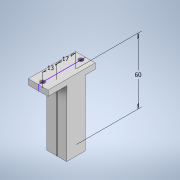
# Autodesk Inventor part: AdaptadorAnycubic
Saved by Autodesk Inventor 2020.3 (Build 243373000, 373)
## iProperties
Created: 2020-08-24
Part Number: AdaptadorAnycubic
Material: Generic
Document SubType Name: Modeling
Designer: mifer
Density: 1 g/cm^3
Appearance: Default
Author: mifer
Autodesk Inventor part; units mm, degrees
ref_plane "YZ Plane" through (0, 0, 0) normal (1, 0, 0) x (0, 1, 0)
ref_plane "XZ Plane" through (0, 0, 0) normal (0, 1, 0) x (-1, 0, 0)
ref_plane "XY Plane" through (0, 0, 0) normal (0, 0, 1) x (1, 0, 0)
sketch "Sketch1" plane through (0, 0, 0) normal (1, 0, 0) x (0, 1, 0)
  line L0 (0, 0) -> (-60, 0)
  line L1 (-60, 0) -> (-60, -17)
  line L2 (-60, -17) -> (0, -17)
  line L3 (0, -17) -> (0, 0)
  line L4 (0, -22) -> (5, -22)
  line L5 (5, -22) -> (5, 13)
  line L6 (5, 13) -> (0, 13)
  line L7 (0, 13) -> (0, -22)
  line L8 (5, 13) -> (0, 13)
  line L9 (0, 13) -> (0, 17)
  line L10 (0, 17) -> (5, 17)
  line L11 (5, 17) -> (5, 13)
  line L12 (5, -22) -> (0, -22)
  line L13 (0, -22) -> (0, -26)
  line L14 (0, -26) -> (5, -26)
  line L15 (5, -26) -> (5, -22)
  point P0 (0, 13)
  point P1 (0, -17)
  dimension "d0" = 17
  dimension "d1" = 60
  dimension "d2" = 13
  constraints: 32 end point, 8 parallel, 4 horizontal, 4 perpendicular, 1 point on line
  measures "d0" distance of L2.end L0.start
  measures "d1" distance of L1.end L2.end
  measures "d2" distance of L0.start L6.end
extrude "Extrusion1" add sketch "Sketch1" along normal mid plane 18
sketch "Sketch2" plane through (-9, 5, 17) normal (0, 1, 0) x (1, 0, 0)
  circle A0 centre (9, 39) radius 2
  circle A1 centre (9, 4) radius 2
  point P0 (9, 17)
  dimension "d5" = 4
  dimension "d6" = 4
  constraints: 2 centre point
  measures "d5" diameter of A0
  measures "d6" diameter of A1
extrude "Extrusion2" cut sketch "Sketch2" against normal blind 10
body "Solid1"
